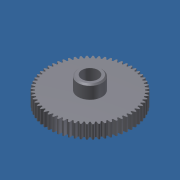
# Autodesk Inventor part: Stirnzahnrad2
Saved by Autodesk Inventor 2014 SP2 (Build 180246200, 246)
## iProperties
Created: 2014-12-14
Part Number: Stirnzahnrad2
Material: Steel
Document SubType Name: Modeling
Designer: 4ndreas
Categories: <?xml version="1.0" encoding="UTF-16"?> <MemberInstance><Categories><FamilyTemplate><FamilyTemplateParameter ValueType="xs:double" Id="1" ObjectReferenceKey="da_z" ObjectType="kUserParameterObject"/><FamilyTemplateParameter ValueType="xs:double" Id="2" ObjectReferenceKey="da_b" ObjectType="kUserParameterObject"/><FamilyTemplateParameter ValueType="xs:double" Id="3" ObjectReferenceKey="da_beta" ObjectType="kUserParameterObject"/><FamilyTemplateParameter ValueType="xs:double" Id="4" ObjectReferenceKey="da_da" ObjectType="kUserParameterObject"/><FamilyTemplateParameter ValueType="xs:double" Id="5" ObjectReferenceKey="da_aw" ObjectType="kUserParameterObject"/><FamilyTemplateParameter ValueType="xs:string" Id="6" ObjectReferenceKey="EAIAABAAAACIAQAAAAAAAIAAAAAAAAAA" ObjectType="83910656" SubObjectId="SurfaceGeometry"/></FamilyTemplate><ParamToTemplateMap><ParamToTemplate CategoryParameter="//CategoryParameter[@InternalName='046C89C9-8512-4d59-83FE-43B91F4F132A']" TemplateParameter="1"/><ParamToTemplate CategoryParameter="//CategoryParameter[@InternalName='2552DF32-E462-4b46-AEBF-C6C7768E72AC']" TemplateParameter="2"/><ParamToTemplate CategoryParameter="//CategoryParameter[@InternalName='C9EE641D-15FC-4fae-A226-E94C4372FDD7']" TemplateParameter="3"/><ParamToTemplate><ParamToTemplate CategoryParameter="//CategoryParameter[@InternalName='00B6519A-459B-49c7-AD84-2E56D39A5744']" ConstantValue="0.402671"/></ParamToTemplate><ParamToTemplate><ParamToTemplate CategoryParameter="//CategoryParameter[@InternalName='04B31F0E-C7A6-4894-AA32-9629BEFACF47']" ConstantValue="1.000000"/></ParamToTemplate><ParamToTemplate><ParamToTemplate CategoryParameter="//CategoryParameter[@InternalName='43CBEC2E-7847-49e7-A936-2F7889FCB2D9']" ConstantValue="0.250000"/></ParamToTemplate><ParamToTemplate><ParamToTemplate CategoryParameter="//CategoryParameter[@InternalName='B1EFC894-105D-4ebd-86BF-FA20ED196853']" ConstantValue="0.350000"/></ParamToTemplate><ParamToTemplate><ParamToTemplate CategoryParameter="//CategoryParameter[@InternalName='51175063-3D10-4879-93E8-6246FE8B403D']" ConstantValue="2060000000.000000"/></ParamToTemplate><ParamToTemplate><ParamToTemplate CategoryParameter="//CategoryParameter[@InternalName='A3A52E27-4454-46a9-B0BD-C932399B70AF']" ConstantValue="0.300000"/></ParamToTemplate><ParamToTemplate><ParamToTemplate CategoryParameter="//CategoryParameter[@InternalName='91B76062-C214-41d9-B1B9-14D2AB99603D']" ConstantValue="0.050000"/></ParamToTemplate><ParamToTemplate><ParamToTemplate CategoryParameter="//CategoryParameter[@InternalName='374E806E-8B8A-4dda-A9AA-1039D6500AD2']" ConstantValue="20.000000"/></ParamToTemplate><ParamToTemplate><ParamToTemplate CategoryParameter="//CategoryParameter[@InternalName='2D373A89-B862-43d6-8D0B-0CBF12AB9F6C']" ConstantValue="0.349066"/></ParamToTemplate><ParamToTemplate CategoryParameter="//CategoryParameter[@InternalName='37777632-D6A2-4fac-9D53-DB8ACD95C989']" TemplateParameter="4"/><ParamToTemplate CategoryParameter="//CategoryParameter[@InternalName='FD1017F1-B727-4f7e-9707-0F86F1FF9423']" TemplateParameter="5"/><ParamToTemplate><ParamToTemplate CategoryParameter="//CategoryParameter[@InternalName='9E1B4470-B2D3-4ff1-B813-535BB4CDF51A']" ConstantValue="3520000.000000"/></ParamToTemplate><ParamToTemplate><ParamToTemplate CategoryParameter="//CategoryParameter[@InternalName='F8452263-BFF6-458c-9FB1-07C4B99E95CD']" ConstantValue="11400000.000000"/></ParamToTemplate><ParamToTemplate><ParamToTemplate CategoryParameter="//CategoryParameter[@InternalName='3E3BB259-FD49-497f-8171-6EBC954A3479']" ConstantValue="2.000000"/></ParamToTemplate><ParamToTemplate CategoryParameter="//CategoryParameter[@InternalName='27C3BAF2-7550-4e4b-AE2C-0DB134B7D9B7']" TemplateParameter="6"/></ParamToTemplateMap><Category DisplayName="Gear" InternalName="DC85795E-93AB-48d5-8EEE-5A27447B64BD" Mnemonic="Gear"><CategoryParameter DisplayName="z" InternalName="046C89C9-8512-4d59-83FE-43B91F4F132A" Mnemonic="z"/><CategoryParameter DisplayName="b" InternalName="2552DF32-E462-4b46-AEBF-C6C7768E72AC" Mnemonic="b"/><CategoryParameter DisplayName="||b|" InternalName="C9EE641D-15FC-4fae-A226-E94C4372FDD7" Mnemonic="beta"/><CategoryParameter DisplayName="x" InternalName="00B6519A-459B-49c7-AD84-2E56D39A5744" Mnemonic="x"/><CategoryParameter DisplayName="a*" InternalName="04B31F0E-C7A6-4894-AA32-9629BEFACF47" Mnemonic="a"/><CategoryParameter DisplayName="c*" InternalName="43CBEC2E-7847-49e7-A936-2F7889FCB2D9" Mnemonic="c"/><CategoryParameter DisplayName="r|.f|*" InternalName="B1EFC894-105D-4ebd-86BF-FA20ED196853" Mnemonic="rf"/><CategoryParameter DisplayName="E" InternalName="51175063-3D10-4879-93E8-6246FE8B403D" Mnemonic="E"/><CategoryParameter DisplayName="||m|" InternalName="A3A52E27-4454-46a9-B0BD-C932399B70AF" Mnemonic="mi"/><Category DisplayName="SpurGear" InternalName="26C5A22E-A91E-4dfd-A3B3-23CCAFAE1764" Mnemonic="SpurGear"><CategoryParameter DisplayName="m" InternalName="91B76062-C214-41d9-B1B9-14D2AB99603D" Mnemonic="m"/><CategoryParameter DisplayName="P" InternalName="374E806E-8B8A-4dda-A9AA-1039D6500AD2" Mnemonic="PP"/><CategoryParameter DisplayName="||a|" InternalName="2D373A89-B862-43d6-8D0B-0CBF12AB9F6C" Mnemonic="alpha"/><CategoryParameter DisplayName="d|.a|" InternalName="37777632-D6A2-4fac-9D53-DB8ACD95C989" Mnemonic="da"/><CategoryParameter DisplayName="a|.w|" InternalName="FD1017F1-B727-4f7e-9707-0F86F1FF9423" Mnemonic="aw"/><CategoryParameter DisplayName="||s||.Flim|" InternalName="9E1B4470-B2D3-4ff1-B813-535BB4CDF51A" Mnemonic="sFlim"/><CategoryParameter DisplayName="||s||.Hlim|" InternalName="F8452263-BFF6-458c-9FB1-07C4B99E95CD" Mnemonic="sHlim"/><CategoryParameter DisplayName="Typ" InternalName="3E3BB259-FD49-497f-8171-6EBC954A3479" Mnemonic="type"/><CategoryParameter DisplayName="PitchDiameter" InternalName="27C3BAF2-7550-4e4b-AE2C-0DB134B7D9B7" Mnemonic="IDS_PITCHDIAM"/></Category></Category></Categories></MemberInstance>
Density: 7.85 g/cm^3
Appearance: Steel
Mass: 28.6034 g
Surface Area: 26.6035 cm^2
Volume: 3.64374 cm^3
CustomPartVersion: 1
Author: 4ndreas
Autodesk Inventor part; units mm, degrees
sketch "Sketch1" plane through (0, 0, 0) normal (0, 0, 1) x (1, 0, 0)
  circle A0 centre (0, 0) radius 15.6951
  dimension "d0" = 31.3903
  constraints: 1 centre point
  measures "d0" diameter of A0
extrude "Extrusion1" add sketch "Sketch1" along normal blind 5
ref_plane "Work Plane2" through (0, 0, 2.5) normal (0, 0, 1) x (1, 0, 0)
sketch "Sketch2" plane through (0, 0, 0) normal (0, 0, -1) x (-1, 0, 0)
  circle A0 centre (0, 0) radius 15.6951 projected
  circle A1 centre (0, 0) radius 15.1301
  dimension "d3" = 30.2602
  constraints: 1 centre point, 1 coincident
  measures "d3" diameter of A1
surface extrude "Flankendurchmesser" sketch "Sketch2" against normal through all shown no curves A1
ref_plane "Work Plane8" through (0, 0, 0) normal (0.9986295, 0.052336, 0) x (0, 0, 1)
ref_plane "Work Plane9" through (0, 0, 0) normal (1, 0, 0) x (0, 1, 0)
spur gear teeth "Stirnzahnrad" teeth 60 pitch diameter 30 tip diameter 31.3903 root diameter 29.1527 face width 5 start plane through (0, 0, 0) normal (0, 0, -1) x (-1, 0, 0)
sketch "Skizze3" plane through (0, 0, 5) normal (0, 0, 1) x (1, 0, 0)
  arc A0 (2.4685, 14.3658) -> (2.0916, 14.4255) centre (0, 0) ccw
  circle A1 centre (0, 0) radius 4.5
  arc A2 (-1.8448, 15.5863) -> (-2.0916, 14.4255) centre (4.0922, 13.7173) ccw projected
  arc A3 (-2.0916, 14.4255) -> (-2.4685, 14.3658) centre (0, 0) ccw projected
  arc A4 (-2.4685, 14.3658) -> (-3.062, 15.3936) centre (-8.1308, 11.7814) ccw projected
  arc A5 (-3.062, 15.3936) -> (-3.4639, 15.3081) centre (0, 0) ccw projected
  arc A6 (-3.4639, 15.3081) -> (-3.588, 14.1278) centre (2.6359, 14.0699) ccw projected
  arc A7 (-3.588, 14.1278) -> (-3.9566, 14.0291) centre (0, 0) ccw projected
  arc A8 (-3.9566, 14.0291) -> (-4.6543, 14.9892) centre (-9.3177, 10.867) ccw projected
  arc A9 (-4.6543, 14.9892) -> (-5.045, 14.8622) centre (0, 0) ccw projected
  arc A10 (-5.045, 14.8622) -> (-5.0451, 13.6754) centre (1.1508, 14.2684) ccw projected
  arc A11 (-5.0451, 13.6754) -> (-5.4014, 13.5386) centre (0, 0) ccw projected
  arc A12 (-5.4014, 13.5386) -> (-6.1956, 14.4206) centre (-10.4026, 9.8335) ccw projected
  arc A13 (-6.1956, 14.4206) -> (-6.5709, 14.2534) centre (0, 0) ccw projected
  arc A14 (-6.5709, 14.2534) -> (-6.4469, 13.0731) centre (-0.347, 14.3105) ccw projected
  arc A15 (-6.4469, 13.0731) -> (-6.787, 12.8999) centre (0, 0) ccw projected
  arc A16 (-6.787, 12.8999) -> (-7.669, 13.6939) centre (-11.3735, 8.6922) ccw projected
  arc A17 (-7.669, 13.6939) -> (-8.0248, 13.4885) centre (0, 0) ccw projected
  arc A18 (-8.0248, 13.4885) -> (-7.7781, 12.3276) centre (-1.841, 14.1958) ccw projected
  arc A19 (-7.7781, 12.3276) -> (-8.0982, 12.1198) centre (0, 0) ccw projected
  arc A20 (-8.0982, 12.1198) -> (-9.0584, 12.8173) centre (-12.2197, 7.4558) ccw projected
  arc A21 (-9.0584, 12.8173) -> (-9.3908, 12.5758) centre (0, 0) ccw projected
  arc A22 (-9.3908, 12.5758) -> (-9.0241, 11.447) centre (-3.3147, 13.9256) ccw projected
  arc A23 (-9.0241, 11.447) -> (-9.3207, 11.2069) centre (0, 0) ccw projected
  arc A24 (-9.3207, 11.2069) -> (-10.3485, 11.8002) centre (-12.9321, 6.1376) ccw projected
  arc A25 (-10.3485, 11.8002) -> (-10.6539, 11.5253) centre (0, 0) ccw projected
  arc A26 (-10.6539, 11.5253) -> (-10.1712, 10.4411) centre (-4.7522, 13.5028) ccw projected
  arc A27 (-10.1712, 10.4411) -> (-10.4411, 10.1712) centre (0, 0) ccw projected
  arc A28 (-10.4411, 10.1712) -> (-11.5253, 10.6539) centre (-13.5028, 4.7522) ccw projected
  arc A29 (-11.5253, 10.6539) -> (-11.8002, 10.3485) centre (0, 0) ccw projected
  arc A30 (-11.8002, 10.3485) -> (-11.2069, 9.3207) centre (-6.1376, 12.9321) ccw projected
  arc A31 (-11.2069, 9.3207) -> (-11.447, 9.0241) centre (0, 0) ccw projected
  arc A32 (-11.447, 9.0241) -> (-12.5758, 9.3908) centre (-13.9256, 3.3147) ccw projected
  arc A33 (-12.5758, 9.3908) -> (-12.8173, 9.0584) centre (0, 0) ccw projected
  arc A34 (-12.8173, 9.0584) -> (-12.1198, 8.0982) centre (-7.4558, 12.2197) ccw projected
  arc A35 (-12.1198, 8.0982) -> (-12.3276, 7.7781) centre (0, 0) ccw projected
  arc A36 (-12.3276, 7.7781) -> (-13.4885, 8.0248) centre (-14.1958, 1.841) ccw projected
  arc A37 (-13.4885, 8.0248) -> (-13.6939, 7.669) centre (0, 0) ccw projected
  arc A38 (-13.6939, 7.669) -> (-12.8999, 6.787) centre (-8.6922, 11.3735) ccw projected
  arc A39 (-12.8999, 6.787) -> (-13.0731, 6.4469) centre (0, 0) ccw projected
  arc A40 (-13.0731, 6.4469) -> (-14.2534, 6.5709) centre (-14.3105, 0.347) ccw projected
  arc A41 (-14.2534, 6.5709) -> (-14.4206, 6.1956) centre (0, 0) ccw projected
  arc A42 (-14.4206, 6.1956) -> (-13.5386, 5.4014) centre (-9.8335, 10.4026) ccw projected
  arc A43 (-13.5386, 5.4014) -> (-13.6754, 5.0451) centre (0, 0) ccw projected
  arc A44 (-13.6754, 5.0451) -> (-14.8622, 5.045) centre (-14.2684, -1.1508) ccw projected
  arc A45 (-14.8622, 5.045) -> (-14.9892, 4.6543) centre (0, 0) ccw projected
  arc A46 (-14.9892, 4.6543) -> (-14.0291, 3.9566) centre (-10.867, 9.3177) ccw projected
  arc A47 (-14.0291, 3.9566) -> (-14.1278, 3.588) centre (0, 0) ccw projected
  arc A48 (-14.1278, 3.588) -> (-15.3081, 3.4639) centre (-14.0699, -2.6359) ccw projected
  arc A49 (-15.3081, 3.4639) -> (-15.3936, 3.062) centre (0, 0) ccw projected
  arc A50 (-15.3936, 3.062) -> (-14.3658, 2.4685) centre (-11.7814, 8.1308) ccw projected
  arc A51 (-14.3658, 2.4685) -> (-14.4255, 2.0916) centre (0, 0) ccw projected
  arc A52 (-14.4255, 2.0916) -> (-15.5863, 1.8448) centre (-13.7173, -4.0922) ccw projected
  arc A53 (-15.5863, 1.8448) -> (-15.6293, 1.4361) centre (0, 0) ccw projected
  arc A54 (-15.6293, 1.4361) -> (-14.5451, 0.9533) centre (-12.5667, 6.8547) ccw projected
  arc A55 (-14.5451, 0.9533) -> (-14.5651, 0.5723) centre (0, 0) ccw projected
  arc A56 (-14.5651, 0.5723) -> (-15.6938, 0.2054) centre (-13.2144, -5.5036) ccw projected
  arc A57 (-15.6938, 0.2054) -> (-15.6938, -0.2054) centre (0, 0) ccw projected
  arc A58 (-15.6938, -0.2054) -> (-14.5651, -0.5723) centre (-13.2144, 5.5036) ccw projected
  arc A59 (-14.5651, -0.5723) -> (-14.5451, -0.9533) centre (0, 0) ccw projected
  arc A60 (-14.5451, -0.9533) -> (-15.6293, -1.4361) centre (-12.5667, -6.8547) ccw projected
  arc A61 (-15.6293, -1.4361) -> (-15.5863, -1.8448) centre (0, 0) ccw projected
  arc A62 (-15.5863, -1.8448) -> (-14.4255, -2.0916) centre (-13.7173, 4.0922) ccw projected
  arc A63 (-14.4255, -2.0916) -> (-14.3658, -2.4685) centre (0, 0) ccw projected
  arc A64 (-14.3658, -2.4685) -> (-15.3936, -3.062) centre (-11.7814, -8.1308) ccw projected
  arc A65 (-15.3936, -3.062) -> (-15.3081, -3.4639) centre (0, 0) ccw projected
  arc A66 (-15.3081, -3.4639) -> (-14.1278, -3.588) centre (-14.0699, 2.6359) ccw projected
  arc A67 (-14.1278, -3.588) -> (-14.0291, -3.9566) centre (0, 0) ccw projected
  arc A68 (-14.0291, -3.9566) -> (-14.9892, -4.6543) centre (-10.867, -9.3177) ccw projected
  arc A69 (-14.9892, -4.6543) -> (-14.8622, -5.045) centre (0, 0) ccw projected
  arc A70 (-14.8622, -5.045) -> (-13.6754, -5.0451) centre (-14.2684, 1.1508) ccw projected
  arc A71 (-13.6754, -5.0451) -> (-13.5386, -5.4014) centre (0, 0) ccw projected
  arc A72 (-13.5386, -5.4014) -> (-14.4206, -6.1956) centre (-9.8335, -10.4026) ccw projected
  arc A73 (-14.4206, -6.1956) -> (-14.2534, -6.5709) centre (0, 0) ccw projected
  arc A74 (-14.2534, -6.5709) -> (-13.0731, -6.4469) centre (-14.3105, -0.347) ccw projected
  arc A75 (-13.0731, -6.4469) -> (-12.8999, -6.787) centre (0, 0) ccw projected
  arc A76 (-12.8999, -6.787) -> (-13.6939, -7.669) centre (-8.6922, -11.3735) ccw projected
  arc A77 (-13.6939, -7.669) -> (-13.4885, -8.0248) centre (0, 0) ccw projected
  arc A78 (-13.4885, -8.0248) -> (-12.3276, -7.7781) centre (-14.1958, -1.841) ccw projected
  arc A79 (-12.3276, -7.7781) -> (-12.1198, -8.0982) centre (0, 0) ccw projected
  arc A80 (-12.1198, -8.0982) -> (-12.8173, -9.0584) centre (-7.4558, -12.2197) ccw projected
  arc A81 (-12.8173, -9.0584) -> (-12.5758, -9.3908) centre (0, 0) ccw projected
  arc A82 (-12.5758, -9.3908) -> (-11.447, -9.0241) centre (-13.9256, -3.3147) ccw projected
  arc A83 (-11.447, -9.0241) -> (-11.2069, -9.3207) centre (0, 0) ccw projected
  arc A84 (-11.2069, -9.3207) -> (-11.8002, -10.3485) centre (-6.1376, -12.9321) ccw projected
  arc A85 (-11.8002, -10.3485) -> (-11.5253, -10.6539) centre (0, 0) ccw projected
  arc A86 (-11.5253, -10.6539) -> (-10.4411, -10.1712) centre (-13.5028, -4.7522) ccw projected
  arc A87 (-10.4411, -10.1712) -> (-10.1712, -10.4411) centre (0, 0) ccw projected
  arc A88 (-10.1712, -10.4411) -> (-10.6539, -11.5253) centre (-4.7522, -13.5028) ccw projected
  arc A89 (-10.6539, -11.5253) -> (-10.3485, -11.8002) centre (0, 0) ccw projected
  arc A90 (-10.3485, -11.8002) -> (-9.3207, -11.2069) centre (-12.9321, -6.1376) ccw projected
  arc A91 (-9.3207, -11.2069) -> (-9.0241, -11.447) centre (0, 0) ccw projected
  arc A92 (-9.0241, -11.447) -> (-9.3908, -12.5758) centre (-3.3147, -13.9256) ccw projected
  arc A93 (-9.3908, -12.5758) -> (-9.0584, -12.8173) centre (0, 0) ccw projected
  arc A94 (-9.0584, -12.8173) -> (-8.0982, -12.1198) centre (-12.2197, -7.4558) ccw projected
  arc A95 (-8.0982, -12.1198) -> (-7.7781, -12.3276) centre (0, 0) ccw projected
  arc A96 (-7.7781, -12.3276) -> (-8.0248, -13.4885) centre (-1.841, -14.1958) ccw projected
  arc A97 (-8.0248, -13.4885) -> (-7.669, -13.6939) centre (0, 0) ccw projected
  arc A98 (-7.669, -13.6939) -> (-6.787, -12.8999) centre (-11.3735, -8.6922) ccw projected
  arc A99 (-6.787, -12.8999) -> (-6.4469, -13.0731) centre (0, 0) ccw projected
  arc A100 (-6.4469, -13.0731) -> (-6.5709, -14.2534) centre (-0.347, -14.3105) ccw projected
  arc A101 (-6.5709, -14.2534) -> (-6.1956, -14.4206) centre (0, 0) ccw projected
  arc A102 (-6.1956, -14.4206) -> (-5.4014, -13.5386) centre (-10.4026, -9.8335) ccw projected
  arc A103 (-5.4014, -13.5386) -> (-5.0451, -13.6754) centre (0, 0) ccw projected
  arc A104 (-5.0451, -13.6754) -> (-5.045, -14.8622) centre (1.1508, -14.2684) ccw projected
  arc A105 (-5.045, -14.8622) -> (-4.6543, -14.9892) centre (0, 0) ccw projected
  arc A106 (-4.6543, -14.9892) -> (-3.9566, -14.0291) centre (-9.3177, -10.867) ccw projected
  arc A107 (-3.9566, -14.0291) -> (-3.588, -14.1278) centre (0, 0) ccw projected
  arc A108 (-3.588, -14.1278) -> (-3.4639, -15.3081) centre (2.6359, -14.0699) ccw projected
  arc A109 (-3.4639, -15.3081) -> (-3.062, -15.3936) centre (0, 0) ccw projected
  arc A110 (-3.062, -15.3936) -> (-2.4685, -14.3658) centre (-8.1308, -11.7814) ccw projected
  arc A111 (-2.4685, -14.3658) -> (-2.0916, -14.4255) centre (0, 0) ccw projected
  arc A112 (-2.0916, -14.4255) -> (-1.8448, -15.5863) centre (4.0922, -13.7173) ccw projected
  arc A113 (-1.8448, -15.5863) -> (-1.4361, -15.6293) centre (0, 0) ccw projected
  arc A114 (-1.4361, -15.6293) -> (-0.9533, -14.5451) centre (-6.8547, -12.5667) ccw projected
  arc A115 (-0.9533, -14.5451) -> (-0.5723, -14.5651) centre (0, 0) ccw projected
  arc A116 (-0.5723, -14.5651) -> (-0.2054, -15.6938) centre (5.5036, -13.2144) ccw projected
  arc A117 (-0.2054, -15.6938) -> (0.2054, -15.6938) centre (0, 0) ccw projected
  arc A118 (0.2054, -15.6938) -> (0.5723, -14.5651) centre (-5.5036, -13.2144) ccw projected
  arc A119 (0.5723, -14.5651) -> (0.9533, -14.5451) centre (0, 0) ccw projected
  arc A120 (0.9533, -14.5451) -> (1.4361, -15.6293) centre (6.8547, -12.5667) ccw projected
  arc A121 (1.4361, -15.6293) -> (1.8448, -15.5863) centre (0, 0) ccw projected
  arc A122 (1.8448, -15.5863) -> (2.0916, -14.4255) centre (-4.0922, -13.7173) ccw projected
  arc A123 (2.0916, -14.4255) -> (2.4685, -14.3658) centre (0, 0) ccw projected
  arc A124 (2.4685, -14.3658) -> (3.062, -15.3936) centre (8.1308, -11.7814) ccw projected
  arc A125 (3.062, -15.3936) -> (3.4639, -15.3081) centre (0, 0) ccw projected
  arc A126 (3.4639, -15.3081) -> (3.588, -14.1278) centre (-2.6359, -14.0699) ccw projected
  arc A127 (3.588, -14.1278) -> (3.9566, -14.0291) centre (0, 0) ccw projected
  arc A128 (3.9566, -14.0291) -> (4.6543, -14.9892) centre (9.3177, -10.867) ccw projected
  arc A129 (4.6543, -14.9892) -> (5.045, -14.8622) centre (0, 0) ccw projected
  arc A130 (5.045, -14.8622) -> (5.0451, -13.6754) centre (-1.1508, -14.2684) ccw projected
  arc A131 (5.0451, -13.6754) -> (5.4014, -13.5386) centre (0, 0) ccw projected
  arc A132 (5.4014, -13.5386) -> (6.1956, -14.4206) centre (10.4026, -9.8335) ccw projected
  arc A133 (6.1956, -14.4206) -> (6.5709, -14.2534) centre (0, 0) ccw projected
  arc A134 (6.5709, -14.2534) -> (6.4469, -13.0731) centre (0.347, -14.3105) ccw projected
  arc A135 (6.4469, -13.0731) -> (6.787, -12.8999) centre (0, 0) ccw projected
  arc A136 (6.787, -12.8999) -> (7.669, -13.6939) centre (11.3735, -8.6922) ccw projected
  arc A137 (7.669, -13.6939) -> (8.0248, -13.4885) centre (0, 0) ccw projected
  arc A138 (8.0248, -13.4885) -> (7.7781, -12.3276) centre (1.841, -14.1958) ccw projected
  arc A139 (7.7781, -12.3276) -> (8.0982, -12.1198) centre (0, 0) ccw projected
  arc A140 (8.0982, -12.1198) -> (9.0584, -12.8173) centre (12.2197, -7.4558) ccw projected
  arc A141 (9.0584, -12.8173) -> (9.3908, -12.5758) centre (0, 0) ccw projected
  arc A142 (9.3908, -12.5758) -> (9.0241, -11.447) centre (3.3147, -13.9256) ccw projected
  arc A143 (9.0241, -11.447) -> (9.3207, -11.2069) centre (0, 0) ccw projected
  arc A144 (9.3207, -11.2069) -> (10.3485, -11.8002) centre (12.9321, -6.1376) ccw projected
  arc A145 (10.3485, -11.8002) -> (10.6539, -11.5253) centre (0, 0) ccw projected
  arc A146 (10.6539, -11.5253) -> (10.1712, -10.4411) centre (4.7522, -13.5028) ccw projected
  arc A147 (10.1712, -10.4411) -> (10.4411, -10.1712) centre (0, 0) ccw projected
  arc A148 (10.4411, -10.1712) -> (11.5253, -10.6539) centre (13.5028, -4.7522) ccw projected
  arc A149 (11.5253, -10.6539) -> (11.8002, -10.3485) centre (0, 0) ccw projected
  arc A150 (11.8002, -10.3485) -> (11.2069, -9.3207) centre (6.1376, -12.9321) ccw projected
  arc A151 (11.2069, -9.3207) -> (11.447, -9.0241) centre (0, 0) ccw projected
  arc A152 (11.447, -9.0241) -> (12.5758, -9.3908) centre (13.9256, -3.3147) ccw projected
  arc A153 (12.5758, -9.3908) -> (12.8173, -9.0584) centre (0, 0) ccw projected
  arc A154 (12.8173, -9.0584) -> (12.1198, -8.0982) centre (7.4558, -12.2197) ccw projected
  arc A155 (12.1198, -8.0982) -> (12.3276, -7.7781) centre (0, 0) ccw projected
  arc A156 (12.3276, -7.7781) -> (13.4885, -8.0248) centre (14.1958, -1.841) ccw projected
  arc A157 (13.4885, -8.0248) -> (13.6939, -7.669) centre (0, 0) ccw projected
  arc A158 (13.6939, -7.669) -> (12.8999, -6.787) centre (8.6922, -11.3735) ccw projected
  arc A159 (12.8999, -6.787) -> (13.0731, -6.4469) centre (0, 0) ccw projected
  arc A160 (13.0731, -6.4469) -> (14.2534, -6.5709) centre (14.3105, -0.347) ccw projected
  arc A161 (14.2534, -6.5709) -> (14.4206, -6.1956) centre (0, 0) ccw projected
  arc A162 (14.4206, -6.1956) -> (13.5386, -5.4014) centre (9.8335, -10.4026) ccw projected
  arc A163 (13.5386, -5.4014) -> (13.6754, -5.0451) centre (0, 0) ccw projected
  arc A164 (13.6754, -5.0451) -> (14.8622, -5.045) centre (14.2684, 1.1508) ccw projected
  arc A165 (14.8622, -5.045) -> (14.9892, -4.6543) centre (0, 0) ccw projected
  arc A166 (14.9892, -4.6543) -> (14.0291, -3.9566) centre (10.867, -9.3177) ccw projected
  arc A167 (14.0291, -3.9566) -> (14.1278, -3.588) centre (0, 0) ccw projected
  arc A168 (14.1278, -3.588) -> (15.3081, -3.4639) centre (14.0699, 2.6359) ccw projected
  arc A169 (15.3081, -3.4639) -> (15.3936, -3.062) centre (0, 0) ccw projected
  arc A170 (15.3936, -3.062) -> (14.3658, -2.4685) centre (11.7814, -8.1308) ccw projected
  arc A171 (14.3658, -2.4685) -> (14.4255, -2.0916) centre (0, 0) ccw projected
  arc A172 (14.4255, -2.0916) -> (15.5863, -1.8448) centre (13.7173, 4.0922) ccw projected
  arc A173 (15.5863, -1.8448) -> (15.6293, -1.4361) centre (0, 0) ccw projected
  arc A174 (15.6293, -1.4361) -> (14.5451, -0.9533) centre (12.5667, -6.8547) ccw projected
  arc A175 (14.5451, -0.9533) -> (14.5651, -0.5723) centre (0, 0) ccw projected
  arc A176 (14.5651, -0.5723) -> (15.6938, -0.2054) centre (13.2144, 5.5036) ccw projected
  arc A177 (15.6938, -0.2054) -> (15.6938, 0.2054) centre (0, 0) ccw projected
  arc A178 (15.6938, 0.2054) -> (14.5651, 0.5723) centre (13.2144, -5.5036) ccw projected
  arc A179 (14.5651, 0.5723) -> (14.5451, 0.9533) centre (0, 0) ccw projected
  arc A180 (14.5451, 0.9533) -> (15.6293, 1.4361) centre (12.5667, 6.8547) ccw projected
  arc A181 (15.6293, 1.4361) -> (15.5863, 1.8448) centre (0, 0) ccw projected
  arc A182 (15.5863, 1.8448) -> (14.4255, 2.0916) centre (13.7173, -4.0922) ccw projected
  arc A183 (14.4255, 2.0916) -> (14.3658, 2.4685) centre (0, 0) ccw projected
  arc A184 (14.3658, 2.4685) -> (15.3936, 3.062) centre (11.7814, 8.1308) ccw projected
  arc A185 (15.3936, 3.062) -> (15.3081, 3.4639) centre (0, 0) ccw projected
  arc A186 (15.3081, 3.4639) -> (14.1278, 3.588) centre (14.0699, -2.6359) ccw projected
  arc A187 (14.1278, 3.588) -> (14.0291, 3.9566) centre (0, 0) ccw projected
  arc A188 (14.0291, 3.9566) -> (14.9892, 4.6543) centre (10.867, 9.3177) ccw projected
  arc A189 (14.9892, 4.6543) -> (14.8622, 5.045) centre (0, 0) ccw projected
  arc A190 (14.8622, 5.045) -> (13.6754, 5.0451) centre (14.2684, -1.1508) ccw projected
  arc A191 (13.6754, 5.0451) -> (13.5386, 5.4014) centre (0, 0) ccw projected
  arc A192 (13.5386, 5.4014) -> (14.4206, 6.1956) centre (9.8335, 10.4026) ccw projected
  arc A193 (14.4206, 6.1956) -> (14.2534, 6.5709) centre (0, 0) ccw projected
  arc A194 (14.2534, 6.5709) -> (13.0731, 6.4469) centre (14.3105, 0.347) ccw projected
  arc A195 (13.0731, 6.4469) -> (12.8999, 6.787) centre (0, 0) ccw projected
  arc A196 (12.8999, 6.787) -> (13.6939, 7.669) centre (8.6922, 11.3735) ccw projected
  arc A197 (13.6939, 7.669) -> (13.4885, 8.0248) centre (0, 0) ccw projected
  arc A198 (13.4885, 8.0248) -> (12.3276, 7.7781) centre (14.1958, 1.841) ccw projected
  arc A199 (12.3276, 7.7781) -> (12.1198, 8.0982) centre (0, 0) ccw projected
  arc A200 (12.1198, 8.0982) -> (12.8173, 9.0584) centre (7.4558, 12.2197) ccw projected
  arc A201 (12.8173, 9.0584) -> (12.5758, 9.3908) centre (0, 0) ccw projected
  arc A202 (12.5758, 9.3908) -> (11.447, 9.0241) centre (13.9256, 3.3147) ccw projected
  arc A203 (11.447, 9.0241) -> (11.2069, 9.3207) centre (0, 0) ccw projected
  arc A204 (11.2069, 9.3207) -> (11.8002, 10.3485) centre (6.1376, 12.9321) ccw projected
  arc A205 (11.8002, 10.3485) -> (11.5253, 10.6539) centre (0, 0) ccw projected
  arc A206 (11.5253, 10.6539) -> (10.4411, 10.1712) centre (13.5028, 4.7522) ccw projected
  arc A207 (10.4411, 10.1712) -> (10.1712, 10.4411) centre (0, 0) ccw projected
  arc A208 (10.1712, 10.4411) -> (10.6539, 11.5253) centre (4.7522, 13.5028) ccw projected
  arc A209 (10.6539, 11.5253) -> (10.3485, 11.8002) centre (0, 0) ccw projected
  arc A210 (10.3485, 11.8002) -> (9.3207, 11.2069) centre (12.9321, 6.1376) ccw projected
  arc A211 (9.3207, 11.2069) -> (9.0241, 11.447) centre (0, 0) ccw projected
  arc A212 (9.0241, 11.447) -> (9.3908, 12.5758) centre (3.3147, 13.9256) ccw projected
  arc A213 (9.3908, 12.5758) -> (9.0584, 12.8173) centre (0, 0) ccw projected
  arc A214 (9.0584, 12.8173) -> (8.0982, 12.1198) centre (12.2197, 7.4558) ccw projected
  arc A215 (8.0982, 12.1198) -> (7.7781, 12.3276) centre (0, 0) ccw projected
  arc A216 (7.7781, 12.3276) -> (8.0248, 13.4885) centre (1.841, 14.1958) ccw projected
  arc A217 (8.0248, 13.4885) -> (7.669, 13.6939) centre (0, 0) ccw projected
  arc A218 (7.669, 13.6939) -> (6.787, 12.8999) centre (11.3735, 8.6922) ccw projected
  arc A219 (6.787, 12.8999) -> (6.4469, 13.0731) centre (0, 0) ccw projected
  arc A220 (6.4469, 13.0731) -> (6.5709, 14.2534) centre (0.347, 14.3105) ccw projected
  arc A221 (6.5709, 14.2534) -> (6.1956, 14.4206) centre (0, 0) ccw projected
  arc A222 (6.1956, 14.4206) -> (5.4014, 13.5386) centre (10.4026, 9.8335) ccw projected
  arc A223 (5.4014, 13.5386) -> (5.0451, 13.6754) centre (0, 0) ccw projected
  arc A224 (5.0451, 13.6754) -> (5.045, 14.8622) centre (-1.1508, 14.2684) ccw projected
  arc A225 (5.045, 14.8622) -> (4.6543, 14.9892) centre (0, 0) ccw projected
  arc A226 (4.6543, 14.9892) -> (3.9566, 14.0291) centre (9.3177, 10.867) ccw projected
  arc A227 (3.9566, 14.0291) -> (3.588, 14.1278) centre (0, 0) ccw projected
  arc A228 (3.588, 14.1278) -> (3.4639, 15.3081) centre (-2.6359, 14.0699) ccw projected
  arc A229 (3.4639, 15.3081) -> (3.062, 15.3936) centre (0, 0) ccw projected
  arc A230 (3.062, 15.3936) -> (2.4685, 14.3658) centre (8.1308, 11.7814) ccw projected
  arc A231 (2.4685, 14.3658) -> (2.0916, 14.4255) centre (0, 0) ccw projected
  arc A232 (2.0916, 14.4255) -> (1.8448, 15.5863) centre (-4.0922, 13.7173) ccw projected
  arc A233 (1.8448, 15.5863) -> (1.4361, 15.6293) centre (0, 0) ccw projected
  arc A234 (1.4361, 15.6293) -> (0.9533, 14.5451) centre (6.8547, 12.5667) ccw projected
  arc A235 (0.9533, 14.5451) -> (0.5723, 14.5651) centre (0, 0) ccw projected
  arc A236 (0.5723, 14.5651) -> (0.2054, 15.6938) centre (-5.5036, 13.2144) ccw projected
  arc A237 (0.2054, 15.6938) -> (-0.2054, 15.6938) centre (0, 0) ccw projected
  arc A238 (-0.2054, 15.6938) -> (-0.5723, 14.5651) centre (5.5036, 13.2144) ccw projected
  arc A239 (-0.5723, 14.5651) -> (-0.9533, 14.5451) centre (0, 0) ccw projected
  arc A240 (-0.9533, 14.5451) -> (-1.4361, 15.6293) centre (-6.8547, 12.5667) ccw projected
  arc A241 (-1.4361, 15.6293) -> (-1.8448, 15.5863) centre (0, 0) ccw projected
  dimension "d49" = 9
  constraints: 2 centre point, 2 point on circle, 1 coincident
  measures "d49" diameter of A1
extrude "Extrusion2" add sketch "Skizze3" along normal blind 5 contours A1
hole "Bohrung1" at (0, 0, 10) direction (0, 0, -1) diameter 6 end through all
chamfer "Fase1" distance 0.5 angle 45 1 edges at (-4.5, 0, 10)
equation "\"d0\" = da_da"
equation "\"d1\" = da_b"
equation "\"d3\" = da_dw"
equation "\"d16\" = da_aw"
equation "\"d43\" = da_aw"
equation "\"d46\" = da_aw"
equation "\"da_da\" = 31.390267"
equation "\"da_b\" = 5"
equation "\"da_dw\" = 30.260178"
equation "\"da_aw\" = 22.695134"
body "Solid1"
body "Srf1"
